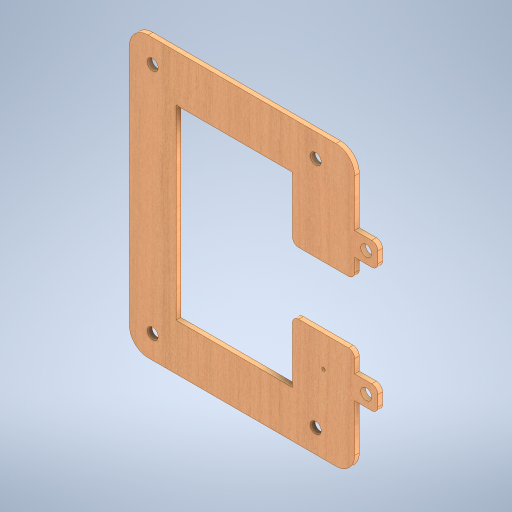
# Autodesk Inventor part: MarcoBC
Saved by Autodesk Inventor 2023.1 (Build 271208000, 208)
## iProperties
Created: 2022-11-11
Part Number: MarcoBC
Material: MDF Medium Density Fiberboard
Document SubType Name: Modeling
Designer: Daniel Peña
Density: 0.8 g/cm^3
Appearance: Cherry - Natural Low Gloss
Author: Daniel Peña
Autodesk Inventor part; units mm, degrees
ref_plane "YZ Plane" through (0, 0, 0) normal (1, 0, 0) x (0, 1, 0)
ref_plane "XZ Plane" through (0, 0, 0) normal (0, 1, 0) x (-1, 0, 0)
ref_plane "XY Plane" through (0, 0, 0) normal (0, 0, 1) x (1, 0, 0)
sketch "Sketch1" plane through (0, 0, 0) normal (0, 0, 1) x (1, 0, 0)
  line L0 (40.11, 59.8927) -> (-34.89, 59.8927)
  line L1 (-34.89, 59.8927) -> (-34.89, -60.1073)
  line L2 (-34.89, -60.1073) -> (40.11, -60.1073)
  line L3 (-52.89, 89.8927) -> (68.11, 89.8927)
  line L4 (68.11, -90.1073) -> (-52.89, -90.1073)
  line L5 (-64.89, -78.1073) -> (-64.89, 77.8927)
  line L6 (80.11, 47.3927) -> (91.11, 47.3927)
  line L7 (95.11, 43.3927) -> (95.11, 36.3927)
  line L8 (91.11, 32.3927) -> (80.11, 32.3927)
  line L9 (115.11, -0.1073) -> (-34.89, -0.1073) construction
  line L10 (80.11, -47.6073) -> (91.11, -47.6073)
  line L11 (95.11, -43.6073) -> (95.11, -36.6073)
  line L12 (91.11, -32.6073) -> (80.11, -32.6073)
  line L13 (80.11, 77.8927) -> (80.11, 47.3927)
  line L14 (80.11, -47.6073) -> (80.11, -78.1073)
  arc A0 (95.11, 43.3927) -> (91.11, 47.3927) centre (91.11, 43.3927) ccw
  arc A1 (91.11, 32.3927) -> (95.11, 36.3927) centre (91.11, 36.3927) ccw
  arc A2 (95.11, -36.6073) -> (91.11, -32.6073) centre (91.11, -36.6073) ccw
  arc A3 (91.11, -47.6073) -> (95.11, -43.6073) centre (91.11, -43.6073) ccw
  arc A4 (80.11, 77.8927) -> (68.11, 89.8927) centre (68.11, 77.8927) ccw
  arc A5 (68.11, -90.1073) -> (80.11, -78.1073) centre (68.11, -78.1073) ccw
  arc A6 (-64.89, -78.1073) -> (-52.89, -90.1073) centre (-52.89, -78.1073) ccw
  arc A7 (-52.89, 89.8927) -> (-64.89, 77.8927) centre (-52.89, 77.8927) ccw
  line L15 (44.11, 19.8927) -> (76.11, 19.8927)
  line L16 (76.11, -20.1073) -> (44.11, -20.1073)
  line L17 (80.11, 32.3927) -> (80.11, 23.8927)
  line L18 (80.11, -24.1073) -> (80.11, -32.6073)
  line L19 (40.11, -60.1073) -> (40.11, -24.1073)
  line L20 (40.11, 23.8927) -> (40.11, 59.8927)
  arc A8 (76.11, 19.8927) -> (80.11, 23.8927) centre (76.11, 23.8927) ccw
  arc A9 (40.11, 23.8927) -> (44.11, 19.8927) centre (44.11, 23.8927) ccw
  arc A10 (44.11, -20.1073) -> (40.11, -24.1073) centre (44.11, -24.1073) ccw
  arc A11 (80.11, -24.1073) -> (76.11, -20.1073) centre (76.11, -24.1073) ccw
  line L21 (211.9676, -294.2124) -> (139.9676, -294.2124)
  line L22 (135.9676, -414.2124) -> (215.9676, -414.2124)
  line L23 (139.9676, -334.2124) -> (211.9676, -334.2124)
  line L24 (215.9676, -374.2124) -> (135.9676, -374.2124)
  line L25 (215.9676, -414.2124) -> (215.9676, -374.2124)
  line L26 (135.9676, -298.2124) -> (135.9676, -330.2124)
  line L27 (135.9676, -374.2124) -> (135.9676, -414.2124)
  line L28 (226.9676, -306.7124) -> (215.9676, -306.7124)
  line L29 (215.9676, -321.7124) -> (226.9676, -321.7124)
  line L30 (230.9676, -317.7124) -> (230.9676, -310.7124)
  line L31 (215.9676, -330.2124) -> (215.9676, -321.7124)
  line L32 (215.9676, -306.7124) -> (215.9676, -298.2124)
  arc A12 (230.9676, -310.7124) -> (226.9676, -306.7124) centre (226.9676, -310.7124) ccw
  arc A13 (226.9676, -321.7124) -> (230.9676, -317.7124) centre (226.9676, -317.7124) ccw
  arc A14 (211.9676, -334.2124) -> (215.9676, -330.2124) centre (211.9676, -330.2124) ccw
  arc A15 (135.9676, -330.2124) -> (139.9676, -334.2124) centre (139.9676, -330.2124) ccw
  arc A16 (139.9676, -294.2124) -> (135.9676, -298.2124) centre (139.9676, -298.2124) ccw
  arc A17 (215.9676, -298.2124) -> (211.9676, -294.2124) centre (211.9676, -298.2124) ccw
  point P0 (95.11, 32.3927)
  point P1 (95.11, 47.3927)
  point P2 (87.61, 39.8927)
  point P3 (87.61, -40.1073)
  point P4 (95.11, -32.6073)
  point P5 (95.11, -47.6073)
  point P6 (87.61, -40.1073)
  point P7 (135.9676, -294.2124)
  point P8 (135.9676, -334.2124)
  point P9 (230.9676, -306.7124)
  dimension "d22" = 75
  dimension "d23" = 120
  dimension "d24" = 30
  dimension "d25" = 15
  dimension "d26" = 15
  dimension "d27" = 80
  dimension "d28" = 4
  dimension "d29" = 4
  dimension "d30" = 12
  dimension "d31" = 40
  dimension "d32" = 4
  dimension "d33" = 7.5
  dimension "d34" = 7.5
  dimension "d52" = 80
  dimension "d53" = 120
  dimension "d54" = 40
  dimension "d55" = 40
  dimension "d56" = 15
  dimension "d58" = 15
  dimension "d59" = 12.5
  dimension "d60" = 12.5
  dimension "d61" = 4
  dimension "d62" = 40
  dimension "d63" = 15
  constraints: 66 end point, 36 point on circle, 36 tangent, 18 centre point, 17 parallel, 14 perpendicular, 14 point on line, 13 equal radius, 6 symmetric about line, 4 horizontal, 1 collinear, 1 midpoint, 2 other
  measures "d22" distance of L2.end L1.end
  measures "d23" distance of L1.end L0.end
  measures "d24" distance between parallel lines of L0 L3
  measures "d25" distance of point (95.11, 32.393) L8.end
  measures "d26" distance of point (95.11, 47.393) point (95.11, 32.393)
  measures "d27" distance of point (87.61, -40.107) point (87.61, 39.893)
  measures "d28" radius of A0
  measures "d29" radius of A2
  measures "d30" radius of A4
  measures "d31" distance between parallel lines of L16 L15
  measures "d32" radius of A8
  measures "d33" distance from line of point (87.61, 39.893) L6
  measures "d34" distance from line of L7 point (87.61, 39.893)
  measures "d52" distance of L22.end L22.start
  measures "d53" distance of L22.start point (135.968, -294.212)
  measures "d54" distance of point (135.968, -294.212) point (135.968, -334.212)
  measures "d55" distance of L22.end L24.start
  measures "d56" distance between parallel lines of L29 L28
  measures "d58" distance of point (230.968, -306.712) L28.end
  measures "d59" distance between parallel lines of L21 L28
  measures "d60" distance between parallel lines of L23 L29
  measures "d61" radius of A12
  measures "d62" distance between parallel lines of L19 L14
  measures "d63" distance between parallel lines of L11 L14
extrude "Extrusion1" add sketch "Sketch1" along normal blind 3 contours L0 L1 L2 L19 A10 L16 A11 L18 L12 A2 L11 A3 L10 L14 A5 L4 A6 L5 A7 L3 A4 L13 L6 A0 L7 A1 L8 L17 A8 L15 A9 L20
sketch "Sketch3" plane through (0, 0, 3) normal (0, 0, 1) x (1, 0, 0)
  line L0 (95.11, 36.3927) -> (95.11, 43.3927) projected
  line L1 (95.11, -43.6073) -> (95.11, -36.6073) projected
  line L2 (91.11, 47.3927) -> (80.11, 47.3927) projected
  point P0 (0, 0)
  point P1 (87.61, 39.8927)
  point P2 (87.61, -40.1073)
  dimension "d35" = 7.5
  dimension "d36" = 7.5
  dimension "d37" = 80
  dimension "d38" = 7.5
  measures "d35" distance from line of L0 point (87.61, 39.893)
  measures "d36" distance from line of L1 point (87.61, -40.107)
  measures "d37" distance of point (87.61, 39.893) point (87.61, -40.107)
  measures "d38" distance from line of L2 point (87.61, 39.893)
hole "Hole1" at (87.61, 39.8927, 3) at (87.61, -40.1073, 3) direction (0, 0, -1) diameter 7 end through all
sketch "Sketch4" plane through (0, 0, 3) normal (0, 0, 1) x (1, 0, 0)
  line L0 (-64.89, 77.8927) -> (-64.89, -78.1073) projected
  line L1 (-64.89, -0.1073) -> (63.4668, -0.1073) construction
  line L2 (-52.89, -90.1073) -> (68.11, -90.1073) projected
  line L3 (68.11, 89.8927) -> (-52.89, 89.8927) projected
  point P0 (0, 0)
  point P1 (-49.89, 74.8927)
  point P2 (-49.89, -75.1073)
  point P3 (55.11, -75.1073)
  point P4 (55.11, 74.8927)
  dimension "d64" = 15
  dimension "d65" = 15
  dimension "d66" = 105
  dimension "d74" = 15
  constraints: 2 end point, 2 symmetric about line, 1 horizontal, 1 midpoint
  measures "d64" distance from line of L0 point (-49.89, -75.107)
  measures "d65" distance from line of point (-49.89, -75.107) L2
  measures "d66" distance of point (55.11, 74.893) point (-49.89, 74.893)
  measures "d74" distance from line of L3 point (55.11, 74.893)
hole "Hole2" at (-49.89, 74.8927, 3) at (-49.89, -75.1073, 3) at (55.11, -75.1073, 3) at (55.11, 74.8927, 3) direction (0, 0, -1) diameter 7 end through all
sketch "Sketch5" plane through (0, 0, 3) normal (0, 0, 1) x (1, 0, 0)
  line L0 (76.11, -20.1073) -> (44.11, -20.1073) projected
  line L1 (40.11, -24.1073) -> (40.11, -60.1073) projected
  point P0 (0, 0)
  point P1 (60.11, -40.1073)
  dimension "d75" = 20
  dimension "d76" = 20
  measures "d75" distance from line of point (60.11, -40.107) L0
  measures "d76" distance from line of L1 point (60.11, -40.107)
hole "Hole3" at (60.11, -40.1073, 3) direction (0, 0, -1) diameter 2 depth 1
equation "\"d59\" = d60"
body "Solid1"
